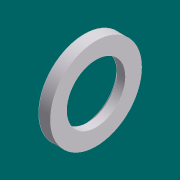
# Autodesk Inventor part: P11
Saved by Autodesk Inventor 2012 SP1 (Build 160190100, 190)
## iProperties
Created: 2011-05-23
Part Number: P11
Material: Aluminium
Document SubType Name: Modeling
Designer: sta
Density: 2.7 g/cm^3
Description: Zentrierring_M1
Mass: 3.51167 g
Surface Area: 12.4281 cm^2
Volume: 1.30062 cm^3
Title: Kart
Author: sta
Autodesk Inventor part; units mm, degrees
ref_plane "YZ Plane" through (0, 0, 0) normal (1, 0, 0) x (0, 1, 0)
ref_plane "XZ Plane" through (0, 0, 0) normal (0, 1, 0) x (-1, 0, 0)
ref_plane "XY Plane" through (0, 0, 0) normal (0, 0, 1) x (1, 0, 0)
sketch "Sketch1" plane through (0, 0, 0) normal (0, 0, 1) x (1, 0, 0)
  line L0 (0, 0) -> (34.0232, 0) construction
  line L1 (0, 0) -> (0, 14)
  line L2 (0, 14) -> (3.6, 14)
  line L3 (3.6, 14) -> (3.6, 0)
  line L4 (3.6, 0) -> (0, 0)
  line L5 (0, 9) -> (3.6, 9)
  dimension "d0" = 18
  dimension "d1" = 28
  dimension "d3" = 3.6
  constraints: 12 end point, 3 point on line, 1 horizontal
  measures "d0" diameter of L5 L0
  measures "d1" diameter of L2 L0
  measures "d3" distance from line of L3 L0.start
revolve "Revolution1" add sketch "Sketch1" angle 360 about axis through (0, 0, 0) along (1, 0, 0) contours L1 L2 L3 L5
chamfer "Chamfer2" distance 1 angle 45 1 edges at (0, -9, 0)
body "Solid1"
